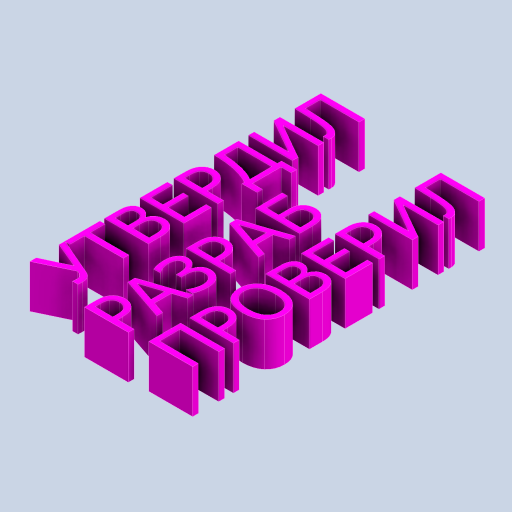
# Autodesk Inventor part: форма
Saved by Autodesk Inventor 2024.2 (Build 282272000, 272)
## iProperties
Created: 2025-11-21
Part Number: форма
Material: Типовые
Document SubType Name: Modeling
Designer: katya_notebook
Density: 1 g/cm^3
Appearance: Пурпурный
Author: katya_notebook
Autodesk Inventor part; units mm, degrees
ref_plane "YZ Plane" through (0, 0, 0) normal (1, 0, 0) x (0, 1, 0)
ref_plane "XZ Plane" through (0, 0, 0) normal (0, 1, 0) x (-1, 0, 0)
ref_plane "XY Plane" through (0, 0, 0) normal (0, 0, 1) x (1, 0, 0)
sketch "Эскиз1" plane through (0, 0, 0) normal (0, 1, 0) x (-1, 0, 0)
  line L0 (9.1599, 8.3568) -> (4.9033, 8.3568)
  line L1 (4.9033, 8.3568) -> (4.9033, -6.3257)
  line L2 (4.9033, -6.3257) -> (9.1599, -6.3257)
  line L3 (9.1599, -6.3257) -> (9.1599, 8.3568)
  line L4 (4.9459, 8.3568) -> (-6.0548, 8.3568)
  line L5 (-6.0548, 8.3568) -> (-6.0548, -6.3257)
  line L6 (-6.0548, -6.3257) -> (4.9459, -6.3257)
  line L7 (4.9459, -6.3257) -> (4.9459, 8.3568)
  line L8 (9.1599, -6.6362) -> (4.9033, -6.6362)
  line L9 (4.9033, -6.6362) -> (4.9033, -20.9369)
  line L10 (4.9033, -20.9369) -> (9.1599, -20.9369)
  line L11 (9.1599, -20.9369) -> (9.1599, -6.6362)
  line L12 (-6.0548, -6.2544) -> (-6.0548, -20.9369)
  line L13 (4.9459, -20.9369) -> (4.9459, -6.6362)
  line L14 (5.8791, -12.5357) -> (5.8791, 8.135)
  line L15 (4.9033, 7.9575) -> (4.9033, -6.7249)
  line L16 (4.9033, -6.7249) -> (9.1599, -6.7249)
  line L17 (9.1599, -6.7249) -> (9.1599, 8.3393)
  line L18 (-6.0548, 8.3393) -> (-6.0548, -6.7249)
  line L19 (4.9459, -6.3432) -> (4.9459, 8.3393)
  line L20 (0.9005, 8.7181) -> (0.9005, -5.6376) construction
  line L21 (0.9005, -5.6376) -> (-2.129, -5.6376) construction
  line L22 (-2.129, -5.6376) -> (-2.129, 8.7181) construction
  line L23 (-2.129, 8.7181) -> (0.9005, 8.7181) construction
  line L24 (-3.3858, 8.5472) -> (-3.3858, -12.3442) construction
  line L25 (-3.3858, -12.3442) -> (-5.6716, -12.3442) construction
  line L26 (-5.6716, -12.3442) -> (-5.6716, 8.5472) construction
  line L27 (-5.6716, 8.5472) -> (-3.3858, 8.5472) construction
  line L28 (5.4799, 7.5583) -> (5.4799, -12.9478) construction
  line L29 (5.4799, -12.9478) -> (1.7428, -12.9478) construction
  line L30 (1.7428, -12.9478) -> (1.7428, 7.5583) construction
  line L31 (1.7428, 7.5583) -> (5.4799, 7.5583) construction
  line L32 (5.4799, 5.1204) -> (2.9136, 6.227)
  spline S0 degree 2 poles (2.9136, 6.227) (2.7505, 6.2961) (2.5554, 6.469) (2.506, 6.5629) knots 0 0 0 1 2 2 2
  spline S1 degree 2 poles (2.506, 6.5629) (2.4541, 6.6592) (2.422, 6.8395) (2.422, 6.9334) knots 0 0 0 1 2 2 2
  spline S2 degree 2 poles (2.422, 6.9334) (2.422, 7.0149) (2.4294, 7.2372) (2.4319, 7.2669) knots 0 0 0 1 2 2 2
  line L33 (2.4319, 7.2669) -> (2.8123, 7.2669)
  line L34 (2.8123, 7.2669) -> (2.8123, 7.2372)
  spline S3 degree 2 poles (2.8123, 7.2372) (2.8073, 7.2076) (2.7975, 7.0816) (2.7975, 6.9853) knots 0 0 0 1 2 2 2
  spline S4 degree 2 poles (2.7975, 6.9853) (2.7975, 6.9408) (2.8073, 6.8173) (2.832, 6.7654) knots 0 0 0 1 2 2 2
  spline S5 degree 2 poles (2.832, 6.7654) (2.8617, 6.7062) (2.9555, 6.6024) (3.0618, 6.5604) knots 0 0 0 1 2 2 2
  line L35 (3.0618, 6.5604) -> (3.2223, 6.4888)
  line L36 (3.2223, 6.4888) -> (5.4799, 7.5608)
  line L37 (5.4799, 7.5608) -> (5.4799, 7.1112)
  line L38 (5.4799, 7.1112) -> (3.6867, 6.2838)
  line L39 (3.6867, 6.2838) -> (5.4799, 5.5378)
  line L40 (5.4799, 5.5378) -> (5.4799, 5.1204)
  line L41 (2.4319, 4.1275) -> (5.1193, 4.1275)
  line L42 (5.1193, 4.1275) -> (5.1193, 5.15)
  line L43 (5.1193, 5.15) -> (5.4799, 5.15)
  line L44 (5.4799, 5.15) -> (5.4799, 2.6998)
  line L45 (5.4799, 2.6998) -> (5.1193, 2.6998)
  line L46 (5.1193, 2.6998) -> (5.1193, 3.7224)
  line L47 (5.1193, 3.7224) -> (2.4319, 3.7224)
  line L48 (2.4319, 3.7224) -> (2.4319, 4.1275)
  spline S6 degree 2 poles (3.368, 0.3236) (3.1408, 0.3236) (2.7925, 0.4965) (2.6789, 0.6398) knots 0 0 0 1 2 2 2
  spline S7 degree 2 poles (2.6789, 0.6398) (2.5455, 0.8127) (2.4319, 1.2054) (2.4319, 1.5167) knots 0 0 0 1 2 2 2
  line L49 (2.4319, 1.5167) -> (2.4319, 2.391)
  line L50 (2.4319, 2.391) -> (5.4799, 2.391)
  line L51 (5.4799, 2.391) -> (5.4799, 1.5833)
  spline S8 degree 2 poles (5.4799, 1.5833) (5.4799, 1.2573) (5.4379, 0.9313) (5.3564, 0.7831) knots 0 0 0 1 2 2 2
  spline S9 degree 2 poles (5.3564, 0.7831) (5.27, 0.6176) (4.9859, 0.4669) (4.7932, 0.4669) knots 0 0 0 1 2 2 2
  spline S10 degree 2 poles (4.7932, 0.4669) (4.5783, 0.4669) (4.2375, 0.6941) (4.1412, 0.8942) knots 0 0 0 1 2 2 2
  line L52 (4.1412, 0.8942) -> (4.1263, 0.8942)
  spline S11 degree 2 poles (4.1263, 0.8942) (4.0522, 0.6225) (3.6595, 0.3236) (3.368, 0.3236) knots 0 0 0 1 2 2 2
  spline S12 degree 2 poles (3.3507, 0.746) (3.5236, 0.746) (3.746, 0.8448) (3.825, 0.993) knots 0 0 0 1 2 2 2
  spline S13 degree 2 poles (3.825, 0.993) (3.8744, 1.0893) (3.904, 1.3166) (3.904, 1.5265) knots 0 0 0 1 2 2 2
  line L53 (3.904, 1.5265) -> (3.904, 1.986)
  line L54 (3.904, 1.986) -> (2.7777, 1.986)
  line L55 (2.7777, 1.986) -> (2.7777, 1.6574)
  spline S14 degree 2 poles (2.7777, 1.6574) (2.7777, 1.3907) (2.8271, 1.0844) (2.9061, 0.9658) knots 0 0 0 1 2 2 2
  spline S15 degree 2 poles (2.9061, 0.9658) (2.9877, 0.8522) (3.1902, 0.746) (3.3507, 0.746) knots 0 0 0 1 2 2 2
  spline S16 degree 2 poles (4.7364, 0.8893) (4.8451, 0.8893) (5.0081, 0.9634) (5.0551, 1.0449) knots 0 0 0 1 2 2 2
  spline S17 degree 2 poles (5.0551, 1.0449) (5.1094, 1.1437) (5.1341, 1.3833) (5.1341, 1.5982) knots 0 0 0 1 2 2 2
  line L56 (5.1341, 1.5982) -> (5.1341, 1.986)
  line L57 (5.1341, 1.986) -> (4.2424, 1.986)
  line L58 (4.2424, 1.986) -> (4.2424, 1.5265)
  spline S18 degree 2 poles (4.2424, 1.5265) (4.2424, 1.3363) (4.2819, 1.156) (4.3437, 1.0597) knots 0 0 0 1 2 2 2
  spline S19 degree 2 poles (4.3437, 1.0597) (4.403, 0.9658) (4.5932, 0.8893) (4.7364, 0.8893) knots 0 0 0 1 2 2 2
  line L59 (2.4319, -0.079) -> (5.4799, -0.079)
  line L60 (5.4799, -0.079) -> (5.4799, -1.9858)
  line L61 (5.4799, -1.9858) -> (5.1193, -1.9858)
  line L62 (5.1193, -1.9858) -> (5.1193, -0.4841)
  line L63 (5.1193, -0.4841) -> (4.2844, -0.4841)
  line L64 (4.2844, -0.4841) -> (4.2844, -1.8846)
  line L65 (4.2844, -1.8846) -> (3.9238, -1.8846)
  line L66 (3.9238, -1.8846) -> (3.9238, -0.4841)
  line L67 (3.9238, -0.4841) -> (2.7925, -0.4841)
  line L68 (2.7925, -0.4841) -> (2.7925, -1.9858)
  line L69 (2.7925, -1.9858) -> (2.4319, -1.9858)
  line L70 (2.4319, -1.9858) -> (2.4319, -0.079)
  spline S20 degree 2 poles (4.5611, -4.357) (4.3635, -4.357) (4.0078, -4.2163) (3.8843, -4.0903) knots 0 0 0 1 2 2 2
  spline S21 degree 2 poles (3.8843, -4.0903) (3.7287, -3.9322) (3.5681, -3.5049) (3.5681, -3.1788) knots 0 0 0 1 2 2 2
  line L71 (3.5681, -3.1788) -> (3.5681, -2.8355)
  line L72 (3.5681, -2.8355) -> (2.4319, -2.8355)
  line L73 (2.4319, -2.8355) -> (2.4319, -2.4304)
  line L74 (2.4319, -2.4304) -> (5.4799, -2.4304)
  line L75 (5.4799, -2.4304) -> (5.4799, -3.1961)
  spline S22 degree 2 poles (5.4799, -3.1961) (5.4799, -3.4678) (5.391, -3.8482) (5.2897, -3.994) knots 0 0 0 1 2 2 2
  spline S23 degree 2 poles (5.2897, -3.994) (5.1736, -4.1644) (4.8155, -4.357) (4.5611, -4.357) knots 0 0 0 1 2 2 2
  spline S24 degree 2 poles (4.5487, -3.9347) (4.7068, -3.9347) (4.939, -3.826) (5.0131, -3.7148) knots 0 0 0 1 2 2 2
  spline S25 degree 2 poles (5.0131, -3.7148) (5.0773, -3.6185) (5.1292, -3.3616) (5.1292, -3.1714) knots 0 0 0 1 2 2 2
  line L76 (5.1292, -3.1714) -> (5.1292, -2.8355)
  line L77 (5.1292, -2.8355) -> (3.9139, -2.8355)
  line L78 (3.9139, -2.8355) -> (3.9139, -3.1122)
  spline S26 degree 2 poles (3.9139, -3.1122) (3.9139, -3.3592) (3.993, -3.663) (4.0967, -3.7618) knots 0 0 0 1 2 2 2
  spline S27 degree 2 poles (4.0967, -3.7618) (4.1881, -3.8532) (4.403, -3.9347) (4.5487, -3.9347) knots 0 0 0 1 2 2 2
  line L79 (1.7428, -7.2173) -> (1.7428, -6.832)
  line L80 (1.7428, -6.832) -> (2.4393, -6.832)
  line L81 (2.4393, -6.832) -> (2.4393, -4.856)
  line L82 (2.4393, -4.856) -> (1.7428, -4.856)
  line L83 (1.7428, -4.856) -> (1.7428, -4.4707)
  line L84 (1.7428, -4.4707) -> (2.7901, -4.4707)
  line L85 (2.7901, -4.4707) -> (2.7901, -4.6362)
  spline S28 degree 2 poles (2.7901, -4.6362) (3.2272, -4.9029) (4.6426, -5.2265) (5.4799, -5.2265) knots 0 0 0 1 2 2 2
  line L86 (5.4799, -5.2265) -> (5.4799, -6.9283)
  line L87 (5.4799, -6.9283) -> (2.7901, -6.9283)
  line L88 (2.7901, -6.9283) -> (2.7901, -7.2173)
  line L89 (2.7901, -7.2173) -> (1.7428, -7.2173)
  line L90 (2.7901, -6.5232) -> (5.1292, -6.5232)
  line L91 (5.1292, -6.5232) -> (5.1292, -5.6044)
  spline S29 degree 2 poles (5.1292, -5.6044) (4.3882, -5.5748) (3.1828, -5.266) (2.7901, -5.0264) knots 0 0 0 1 2 2 2
  line L92 (2.7901, -5.0264) -> (2.7901, -6.5232)
  line L93 (2.4319, -9.7985) -> (2.4319, -9.3934)
  line L94 (2.4319, -9.3934) -> (4.8525, -9.3934)
  line L95 (4.8525, -9.3934) -> (2.4319, -8.0176)
  line L96 (2.4319, -8.0176) -> (2.4319, -7.6076)
  line L97 (2.4319, -7.6076) -> (5.4799, -7.6076)
  line L98 (5.4799, -7.6076) -> (5.4799, -8.0127)
  line L99 (5.4799, -8.0127) -> (3.0988, -8.0127)
  line L100 (3.0988, -8.0127) -> (5.4799, -9.3687)
  line L101 (5.4799, -9.3687) -> (5.4799, -9.7985)
  line L102 (5.4799, -9.7985) -> (2.4319, -9.7985)
  line L103 (2.4319, -12.639) -> (2.4319, -12.2339)
  line L104 (2.4319, -12.2339) -> (5.1193, -12.2339)
  line L105 (5.1193, -12.2339) -> (5.1193, -11.2064)
  spline S30 degree 2 poles (5.1193, -11.2064) (4.8871, -11.2015) (4.4474, -11.1792) (4.2745, -11.1743) knots 0 0 0 1 2 2 2
  spline S31 degree 2 poles (4.2745, -11.1743) (3.8423, -11.157) (3.2791, -11.0854) (3.0889, -11.0286) knots 0 0 0 1 2 2 2
  spline S32 degree 2 poles (3.0889, -11.0286) (2.9012, -10.9717) (2.6715, -10.8235) (2.5949, -10.7346) knots 0 0 0 1 2 2 2
  spline S33 degree 2 poles (2.5949, -10.7346) (2.5109, -10.6432) (2.427, -10.4308) (2.427, -10.2925) knots 0 0 0 1 2 2 2
  spline S34 degree 2 poles (2.427, -10.2925) (2.427, -10.2505) (2.4319, -10.1616) (2.4319, -10.1369) knots 0 0 0 1 2 2 2
  line L106 (2.4319, -10.1369) -> (2.8246, -10.1369)
  line L107 (2.8246, -10.1369) -> (2.8246, -10.1665)
  spline S35 degree 2 poles (2.8246, -10.1665) (2.8222, -10.1863) (2.8197, -10.2159) (2.8197, -10.2431) knots 0 0 0 1 2 2 2
  spline S36 degree 2 poles (2.8197, -10.2431) (2.8197, -10.3172) (2.8642, -10.4432) (2.9111, -10.4901) knots 0 0 0 1 2 2 2
  spline S37 degree 2 poles (2.9111, -10.4901) (3.0494, -10.6284) (3.7509, -10.7569) (4.3437, -10.784) knots 0 0 0 1 2 2 2
  spline S38 degree 2 poles (4.3437, -10.784) (4.5438, -10.7939) (5.2033, -10.8161) (5.4799, -10.8235) knots 0 0 0 1 2 2 2
  line L108 (5.4799, -10.8235) -> (5.4799, -12.639)
  line L109 (5.4799, -12.639) -> (2.4319, -12.639)
  spline S39 degree 2 poles (-0.0727, 6.4827) (-0.2703, 6.4827) (-0.626, 6.6235) (-0.7495, 6.7495) knots 0 0 0 1 2 2 2
  spline S40 degree 2 poles (-0.7495, 6.7495) (-0.9051, 6.9076) (-1.0657, 7.3349) (-1.0657, 7.6609) knots 0 0 0 1 2 2 2
  line L110 (-1.0657, 7.6609) -> (-1.0657, 8.0043)
  line L111 (-1.0657, 8.0043) -> (-2.2019, 8.0043)
  line L112 (-2.2019, 8.0043) -> (-2.2019, 8.4093)
  line L113 (-2.2019, 8.4093) -> (0.8461, 8.4093)
  line L114 (0.8461, 8.4093) -> (0.8461, 7.6436)
  spline S41 degree 2 poles (0.8461, 7.6436) (0.8461, 7.3719) (0.7572, 6.9916) (0.6559, 6.8458) knots 0 0 0 1 2 2 2
  spline S42 degree 2 poles (0.6559, 6.8458) (0.5398, 6.6754) (0.1817, 6.4827) (-0.0727, 6.4827) knots 0 0 0 1 2 2 2
  spline S43 degree 2 poles (-0.0851, 6.9051) (0.073, 6.9051) (0.3052, 7.0138) (0.3793, 7.1249) knots 0 0 0 1 2 2 2
  spline S44 degree 2 poles (0.3793, 7.1249) (0.4435, 7.2213) (0.4954, 7.4782) (0.4954, 7.6683) knots 0 0 0 1 2 2 2
  line L115 (0.4954, 7.6683) -> (0.4954, 8.0043)
  line L116 (0.4954, 8.0043) -> (-0.7199, 8.0043)
  line L117 (-0.7199, 8.0043) -> (-0.7199, 7.7276)
  spline S45 degree 2 poles (-0.7199, 7.7276) (-0.7199, 7.4806) (-0.6408, 7.1768) (-0.5371, 7.078) knots 0 0 0 1 2 2 2
  spline S46 degree 2 poles (-0.5371, 7.078) (-0.4457, 6.9866) (-0.2308, 6.9051) (-0.0851, 6.9051) knots 0 0 0 1 2 2 2
  line L118 (-2.2019, 6.4259) -> (0.8461, 5.3984)
  line L119 (0.8461, 5.3984) -> (0.8461, 4.8995)
  line L120 (0.8461, 4.8995) -> (-2.2019, 3.8719)
  line L121 (-2.2019, 3.8719) -> (-2.2019, 4.2992)
  line L122 (-2.2019, 4.2992) -> (-1.3497, 4.5759)
  line L123 (-1.3497, 4.5759) -> (-1.3497, 5.7393)
  line L124 (-1.3497, 5.7393) -> (-2.2019, 6.0159)
  line L125 (-2.2019, 6.0159) -> (-2.2019, 6.4259)
  line L126 (-1.0039, 4.687) -> (0.4312, 5.1588)
  line L127 (0.4312, 5.1588) -> (-1.0039, 5.6281)
  line L128 (-1.0039, 5.6281) -> (-1.0039, 4.687)
  spline S47 degree 2 poles (-0.7322, 2.0071) (-0.8211, 1.9058) (-1.0854, 1.7724) (-1.2929, 1.7724) knots 0 0 0 1 2 2 2
  spline S48 degree 2 poles (-1.2929, 1.7724) (-1.4979, 1.7724) (-1.8462, 1.9354) (-1.9771, 2.0787) knots 0 0 0 1 2 2 2
  spline S49 degree 2 poles (-1.9771, 2.0787) (-2.113, 2.2269) (-2.2562, 2.6592) (-2.2562, 2.9259) knots 0 0 0 1 2 2 2
  spline S50 degree 2 poles (-2.2562, 2.9259) (-2.2562, 3.21) (-2.1426, 3.6842) (-2.0833, 3.8275) knots 0 0 0 1 2 2 2
  line L129 (-2.0833, 3.8275) -> (-1.6288, 3.8275)
  line L130 (-1.6288, 3.8275) -> (-1.6288, 3.7978)
  spline S51 degree 2 poles (-1.6288, 3.7978) (-1.7375, 3.6348) (-1.903, 3.168) (-1.903, 2.9333) knots 0 0 0 1 2 2 2
  spline S52 degree 2 poles (-1.903, 2.9333) (-1.903, 2.7851) (-1.824, 2.4887) (-1.7326, 2.3874) knots 0 0 0 1 2 2 2
  spline S53 degree 2 poles (-1.7326, 2.3874) (-1.6437, 2.2886) (-1.4337, 2.1948) (-1.2732, 2.1948) knots 0 0 0 1 2 2 2
  spline S54 degree 2 poles (-1.2732, 2.1948) (-1.1175, 2.1948) (-0.9051, 2.3059) (-0.8409, 2.4097) knots 0 0 0 1 2 2 2
  spline S55 degree 2 poles (-0.8409, 2.4097) (-0.7742, 2.5085) (-0.7199, 2.7876) (-0.7199, 2.9457) knots 0 0 0 1 2 2 2
  line L131 (-0.7199, 2.9457) -> (-0.7199, 3.2643)
  line L132 (-0.7199, 3.2643) -> (-0.379, 3.2643)
  line L133 (-0.379, 3.2643) -> (-0.379, 2.9852)
  spline S56 degree 2 poles (-0.379, 2.9852) (-0.379, 2.6641) (-0.1197, 2.2714) (0.1273, 2.2714) knots 0 0 0 1 2 2 2
  spline S57 degree 2 poles (0.1273, 2.2714) (0.241, 2.2714) (0.4015, 2.3677) (0.4534, 2.4541) knots 0 0 0 1 2 2 2
  spline S58 degree 2 poles (0.4534, 2.4541) (0.5077, 2.5505) (0.5472, 2.7629) (0.5472, 2.8864) knots 0 0 0 1 2 2 2
  spline S59 degree 2 poles (0.5472, 2.8864) (0.5472, 3.0173) (0.488, 3.2717) (0.4435, 3.3829) knots 0 0 0 1 2 2 2
  spline S60 degree 2 poles (0.4435, 3.3829) (0.4015, 3.4891) (0.3077, 3.6496) (0.2755, 3.699) knots 0 0 0 1 2 2 2
  line L134 (0.2755, 3.699) -> (0.2755, 3.7262)
  line L135 (0.2755, 3.7262) -> (0.7251, 3.7262)
  spline S61 degree 2 poles (0.7251, 3.7262) (0.7893, 3.5879) (0.9005, 3.1087) (0.9005, 2.8765) knots 0 0 0 1 2 2 2
  spline S62 degree 2 poles (0.9005, 2.8765) (0.9005, 2.6419) (0.8214, 2.301) (0.73, 2.1602) knots 0 0 0 1 2 2 2
  spline S63 degree 2 poles (0.73, 2.1602) (0.6312, 2.0071) (0.3571, 1.8539) (0.1693, 1.8539) knots 0 0 0 1 2 2 2
  spline S64 degree 2 poles (0.1693, 1.8539) (-0.0777, 1.8539) (-0.4457, 2.1824) (-0.505, 2.4492) knots 0 0 0 1 2 2 2
  line L136 (-0.505, 2.4492) -> (-0.5346, 2.4492)
  spline S65 degree 2 poles (-0.5346, 2.4492) (-0.5544, 2.3479) (-0.6482, 2.1083) (-0.7322, 2.0071) knots 0 0 0 1 2 2 2
  spline S66 degree 2 poles (-0.0727, -0.5766) (-0.2703, -0.5766) (-0.626, -0.4358) (-0.7495, -0.3098) knots 0 0 0 1 2 2 2
  spline S67 degree 2 poles (-0.7495, -0.3098) (-0.9051, -0.1517) (-1.0657, 0.2756) (-1.0657, 0.6016) knots 0 0 0 1 2 2 2
  line L137 (-1.0657, 0.6016) -> (-1.0657, 0.945)
  line L138 (-1.0657, 0.945) -> (-2.2019, 0.945)
  line L139 (-2.2019, 0.945) -> (-2.2019, 1.35)
  line L140 (-2.2019, 1.35) -> (0.8461, 1.35)
  line L141 (0.8461, 1.35) -> (0.8461, 0.5843)
  spline S68 degree 2 poles (0.8461, 0.5843) (0.8461, 0.3126) (0.7572, -0.0677) (0.6559, -0.2135) knots 0 0 0 1 2 2 2
  spline S69 degree 2 poles (0.6559, -0.2135) (0.5398, -0.3839) (0.1817, -0.5766) (-0.0727, -0.5766) knots 0 0 0 1 2 2 2
  spline S70 degree 2 poles (-0.0851, -0.1542) (0.073, -0.1542) (0.3052, -0.0455) (0.3793, 0.0656) knots 0 0 0 1 2 2 2
  spline S71 degree 2 poles (0.3793, 0.0656) (0.4435, 0.162) (0.4954, 0.4188) (0.4954, 0.609) knots 0 0 0 1 2 2 2
  line L142 (0.4954, 0.609) -> (0.4954, 0.945)
  line L143 (0.4954, 0.945) -> (-0.7199, 0.945)
  line L144 (-0.7199, 0.945) -> (-0.7199, 0.6683)
  spline S72 degree 2 poles (-0.7199, 0.6683) (-0.7199, 0.4213) (-0.6408, 0.1175) (-0.5371, 0.0187) knots 0 0 0 1 2 2 2
  spline S73 degree 2 poles (-0.5371, 0.0187) (-0.4457, -0.0727) (-0.2308, -0.1542) (-0.0851, -0.1542) knots 0 0 0 1 2 2 2
  line L145 (-2.2019, -0.6334) -> (0.8461, -1.6609)
  line L146 (0.8461, -1.6609) -> (0.8461, -2.1599)
  line L147 (0.8461, -2.1599) -> (-2.2019, -3.1874)
  line L148 (-2.2019, -3.1874) -> (-2.2019, -2.7601)
  line L149 (-2.2019, -2.7601) -> (-1.3497, -2.4834)
  line L150 (-1.3497, -2.4834) -> (-1.3497, -1.32)
  line L151 (-1.3497, -1.32) -> (-2.2019, -1.0434)
  line L152 (-2.2019, -1.0434) -> (-2.2019, -0.6334)
  line L153 (-1.0039, -2.3723) -> (0.4312, -1.9005)
  line L154 (0.4312, -1.9005) -> (-1.0039, -1.4312)
  line L155 (-1.0039, -1.4312) -> (-1.0039, -2.3723)
  spline S74 degree 2 poles (-1.2583, -5.5512) (-1.4782, -5.5512) (-1.8388, -5.3783) (-1.9524, -5.235) knots 0 0 0 1 2 2 2
  spline S75 degree 2 poles (-1.9524, -5.235) (-2.0883, -5.0621) (-2.2019, -4.6694) (-2.2019, -4.3582) knots 0 0 0 1 2 2 2
  line L156 (-2.2019, -4.3582) -> (-2.2019, -3.4764)
  line L157 (-2.2019, -3.4764) -> (0.8461, -3.4764)
  line L158 (0.8461, -3.4764) -> (0.8461, -5.3314)
  line L159 (0.8461, -5.3314) -> (0.4855, -5.3314)
  line L160 (0.4855, -5.3314) -> (0.4855, -3.8815)
  line L161 (0.4855, -3.8815) -> (-0.3494, -3.8815)
  line L162 (-0.3494, -3.8815) -> (-0.3494, -4.3705)
  spline S76 degree 2 poles (-0.3494, -4.3705) (-0.3494, -4.6817) (-0.421, -5.0745) (-0.5569, -5.2474) knots 0 0 0 1 2 2 2
  spline S77 degree 2 poles (-0.5569, -5.2474) (-0.6779, -5.403) (-1.0336, -5.5512) (-1.2583, -5.5512) knots 0 0 0 1 2 2 2
  spline S78 degree 2 poles (-1.2657, -5.1288) (-1.1126, -5.1288) (-0.8804, -5.0275) (-0.8088, -4.9189) knots 0 0 0 1 2 2 2
  spline S79 degree 2 poles (-0.8088, -4.9189) (-0.7322, -4.8077) (-0.7001, -4.5113) (-0.7001, -4.2445) knots 0 0 0 1 2 2 2
  line L163 (-0.7001, -4.2445) -> (-0.7001, -3.8815)
  line L164 (-0.7001, -3.8815) -> (-1.8561, -3.8815)
  line L165 (-1.8561, -3.8815) -> (-1.8561, -4.2347)
  spline S80 degree 2 poles (-1.8561, -4.2347) (-1.8561, -4.5064) (-1.8017, -4.8003) (-1.7276, -4.909) knots 0 0 0 1 2 2 2
  spline S81 degree 2 poles (-1.7276, -4.909) (-1.6486, -5.0251) (-1.4337, -5.1288) (-1.2657, -5.1288) knots 0 0 0 1 2 2 2
  line L166 (-6.498, 6.0254) -> (-6.498, 6.4304)
  line L167 (-6.498, 6.4304) -> (-3.8107, 6.4304)
  line L168 (-3.8107, 6.4304) -> (-3.8107, 7.8334)
  line L169 (-3.8107, 7.8334) -> (-6.498, 7.8334)
  line L170 (-6.498, 7.8334) -> (-6.498, 8.2385)
  line L171 (-6.498, 8.2385) -> (-3.45, 8.2385)
  line L172 (-3.45, 8.2385) -> (-3.45, 6.0254)
  line L173 (-3.45, 6.0254) -> (-6.498, 6.0254)
  spline S82 degree 2 poles (-4.3689, 3.4812) (-4.5665, 3.4812) (-4.9222, 3.622) (-5.0457, 3.748) knots 0 0 0 1 2 2 2
  spline S83 degree 2 poles (-5.0457, 3.748) (-5.2013, 3.9061) (-5.3618, 4.3334) (-5.3618, 4.6594) knots 0 0 0 1 2 2 2
  line L174 (-5.3618, 4.6594) -> (-5.3618, 5.0028)
  line L175 (-5.3618, 5.0028) -> (-6.498, 5.0028)
  line L176 (-6.498, 5.0028) -> (-6.498, 5.4079)
  line L177 (-6.498, 5.4079) -> (-3.45, 5.4079)
  line L178 (-3.45, 5.4079) -> (-3.45, 4.6421)
  spline S84 degree 2 poles (-3.45, 4.6421) (-3.45, 4.3704) (-3.539, 3.9901) (-3.6402, 3.8443) knots 0 0 0 1 2 2 2
  spline S85 degree 2 poles (-3.6402, 3.8443) (-3.7563, 3.6739) (-4.1145, 3.4812) (-4.3689, 3.4812) knots 0 0 0 1 2 2 2
  spline S86 degree 2 poles (-4.3812, 3.9036) (-4.2232, 3.9036) (-3.991, 4.0123) (-3.9169, 4.1234) knots 0 0 0 1 2 2 2
  spline S87 degree 2 poles (-3.9169, 4.1234) (-3.8526, 4.2198) (-3.8008, 4.4767) (-3.8008, 4.6668) knots 0 0 0 1 2 2 2
  line L179 (-3.8008, 4.6668) -> (-3.8008, 5.0028)
  line L180 (-3.8008, 5.0028) -> (-5.016, 5.0028)
  line L181 (-5.016, 5.0028) -> (-5.016, 4.7261)
  spline S88 degree 2 poles (-5.016, 4.7261) (-5.016, 4.4791) (-4.937, 4.1753) (-4.8332, 4.0765) knots 0 0 0 1 2 2 2
  spline S89 degree 2 poles (-4.8332, 4.0765) (-4.7419, 3.9851) (-4.527, 3.9036) (-4.3812, 3.9036) knots 0 0 0 1 2 2 2
  spline S90 degree 2 poles (-3.7983, 0.9396) (-4.0008, 0.7667) (-4.5937, 0.574) (-4.974, 0.574) knots 0 0 0 1 2 2 2
  spline S91 degree 2 poles (-4.974, 0.574) (-5.3445, 0.574) (-5.9448, 0.7618) (-6.1473, 0.9396) knots 0 0 0 1 2 2 2
  spline S92 degree 2 poles (-6.1473, 0.9396) (-6.3597, 1.1273) (-6.5623, 1.6238) (-6.5623, 1.9227) knots 0 0 0 1 2 2 2
  spline S93 degree 2 poles (-6.5623, 1.9227) (-6.5623, 2.2314) (-6.3523, 2.7254) (-6.1473, 2.9057) knots 0 0 0 1 2 2 2
  spline S94 degree 2 poles (-6.1473, 2.9057) (-5.9448, 3.0811) (-5.3495, 3.2688) (-4.974, 3.2688) knots 0 0 0 1 2 2 2
  spline S95 degree 2 poles (-4.974, 3.2688) (-4.5912, 3.2688) (-4.0083, 3.0786) (-3.7983, 2.9033) knots 0 0 0 1 2 2 2
  spline S96 degree 2 poles (-3.7983, 2.9033) (-3.5958, 2.7254) (-3.3858, 2.2289) (-3.3858, 1.9227) knots 0 0 0 1 2 2 2
  spline S97 degree 2 poles (-3.3858, 1.9227) (-3.3858, 1.6114) (-3.6032, 1.1125) (-3.7983, 0.9396) knots 0 0 0 1 2 2 2
  spline S98 degree 2 poles (-4.974, 0.9964) (-4.6727, 0.9964) (-4.2059, 1.1273) (-4.0527, 1.2459) knots 0 0 0 1 2 2 2
  spline S99 degree 2 poles (-4.0527, 1.2459) (-3.8946, 1.3669) (-3.7366, 1.7078) (-3.7366, 1.9202) knots 0 0 0 1 2 2 2
  spline S100 degree 2 poles (-3.7366, 1.9202) (-3.7366, 2.14) (-3.8897, 2.471) (-4.0527, 2.597) knots 0 0 0 1 2 2 2
  spline S101 degree 2 poles (-4.0527, 2.597) (-4.2083, 2.718) (-4.6776, 2.8464) (-4.974, 2.8464) knots 0 0 0 1 2 2 2
  spline S102 degree 2 poles (-4.974, 2.8464) (-5.5743, 2.8464) (-6.2115, 2.3426) (-6.2115, 1.9202) knots 0 0 0 1 2 2 2
  spline S103 degree 2 poles (-6.2115, 1.9202) (-6.2115, 1.4978) (-5.5743, 0.9964) (-4.974, 0.9964) knots 0 0 0 1 2 2 2
  spline S104 degree 2 poles (-5.5619, -1.938) (-5.7891, -1.938) (-6.1374, -1.7651) (-6.251, -1.6218) knots 0 0 0 1 2 2 2
  spline S105 degree 2 poles (-6.251, -1.6218) (-6.3844, -1.4489) (-6.498, -1.0562) (-6.498, -0.745) knots 0 0 0 1 2 2 2
  line L182 (-6.498, -0.745) -> (-6.498, 0.1294)
  line L183 (-6.498, 0.1294) -> (-3.45, 0.1294)
  line L184 (-3.45, 0.1294) -> (-3.45, -0.6783)
  spline S106 degree 2 poles (-3.45, -0.6783) (-3.45, -1.0043) (-3.492, -1.3304) (-3.5735, -1.4786) knots 0 0 0 1 2 2 2
  spline S107 degree 2 poles (-3.5735, -1.4786) (-3.66, -1.644) (-3.944, -1.7947) (-4.1367, -1.7947) knots 0 0 0 1 2 2 2
  spline S108 degree 2 poles (-4.1367, -1.7947) (-4.3516, -1.7947) (-4.6925, -1.5675) (-4.7888, -1.3674) knots 0 0 0 1 2 2 2
  line L185 (-4.7888, -1.3674) -> (-4.8036, -1.3674)
  spline S109 degree 2 poles (-4.8036, -1.3674) (-4.8777, -1.6391) (-5.2704, -1.938) (-5.5619, -1.938) knots 0 0 0 1 2 2 2
  spline S110 degree 2 poles (-5.5792, -1.5156) (-5.4063, -1.5156) (-5.184, -1.4168) (-5.1049, -1.2686) knots 0 0 0 1 2 2 2
  spline S111 degree 2 poles (-5.1049, -1.2686) (-5.0555, -1.1723) (-5.0259, -0.945) (-5.0259, -0.7351) knots 0 0 0 1 2 2 2
  line L186 (-5.0259, -0.7351) -> (-5.0259, -0.2757)
  line L187 (-5.0259, -0.2757) -> (-6.1522, -0.2757)
  line L188 (-6.1522, -0.2757) -> (-6.1522, -0.6042)
  spline S112 degree 2 poles (-6.1522, -0.6042) (-6.1522, -0.8709) (-6.1028, -1.1772) (-6.0238, -1.2958) knots 0 0 0 1 2 2 2
  spline S113 degree 2 poles (-6.0238, -1.2958) (-5.9423, -1.4094) (-5.7397, -1.5156) (-5.5792, -1.5156) knots 0 0 0 1 2 2 2
  spline S114 degree 2 poles (-4.1935, -1.3723) (-4.0848, -1.3723) (-3.9218, -1.2982) (-3.8749, -1.2167) knots 0 0 0 1 2 2 2
  spline S115 degree 2 poles (-3.8749, -1.2167) (-3.8205, -1.1179) (-3.7958, -0.8783) (-3.7958, -0.6634) knots 0 0 0 1 2 2 2
  line L189 (-3.7958, -0.6634) -> (-3.7958, -0.2757)
  line L190 (-3.7958, -0.2757) -> (-4.6875, -0.2757)
  line L191 (-4.6875, -0.2757) -> (-4.6875, -0.7351)
  spline S116 degree 2 poles (-4.6875, -0.7351) (-4.6875, -0.9253) (-4.648, -1.1056) (-4.5862, -1.2019) knots 0 0 0 1 2 2 2
  spline S117 degree 2 poles (-4.5862, -1.2019) (-4.527, -1.2958) (-4.3368, -1.3723) (-4.1935, -1.3723) knots 0 0 0 1 2 2 2
  line L192 (-6.498, -2.3406) -> (-3.45, -2.3406)
  line L193 (-3.45, -2.3406) -> (-3.45, -4.2474)
  line L194 (-3.45, -4.2474) -> (-3.8107, -4.2474)
  line L195 (-3.8107, -4.2474) -> (-3.8107, -2.7457)
  line L196 (-3.8107, -2.7457) -> (-4.6455, -2.7457)
  line L197 (-4.6455, -2.7457) -> (-4.6455, -4.1462)
  line L198 (-4.6455, -4.1462) -> (-5.0061, -4.1462)
  line L199 (-5.0061, -4.1462) -> (-5.0061, -2.7457)
  line L200 (-5.0061, -2.7457) -> (-6.1374, -2.7457)
  line L201 (-6.1374, -2.7457) -> (-6.1374, -4.2474)
  line L202 (-6.1374, -4.2474) -> (-6.498, -4.2474)
  line L203 (-6.498, -4.2474) -> (-6.498, -2.3406)
  spline S118 degree 2 poles (-4.3689, -6.6187) (-4.5665, -6.6187) (-4.9222, -6.4779) (-5.0457, -6.3519) knots 0 0 0 1 2 2 2
  spline S119 degree 2 poles (-5.0457, -6.3519) (-5.2013, -6.1938) (-5.3618, -5.7665) (-5.3618, -5.4405) knots 0 0 0 1 2 2 2
  line L204 (-5.3618, -5.4405) -> (-5.3618, -5.0971)
  line L205 (-5.3618, -5.0971) -> (-6.498, -5.0971)
  line L206 (-6.498, -5.0971) -> (-6.498, -4.692)
  line L207 (-6.498, -4.692) -> (-3.45, -4.692)
  line L208 (-3.45, -4.692) -> (-3.45, -5.4577)
  spline S120 degree 2 poles (-3.45, -5.4577) (-3.45, -5.7294) (-3.539, -6.1098) (-3.6402, -6.2556) knots 0 0 0 1 2 2 2
  spline S121 degree 2 poles (-3.6402, -6.2556) (-3.7563, -6.426) (-4.1145, -6.6187) (-4.3689, -6.6187) knots 0 0 0 1 2 2 2
  spline S122 degree 2 poles (-4.3812, -6.1963) (-4.2232, -6.1963) (-3.991, -6.0876) (-3.9169, -5.9765) knots 0 0 0 1 2 2 2
  spline S123 degree 2 poles (-3.9169, -5.9765) (-3.8526, -5.8801) (-3.8008, -5.6232) (-3.8008, -5.433) knots 0 0 0 1 2 2 2
  line L209 (-3.8008, -5.433) -> (-3.8008, -5.0971)
  line L210 (-3.8008, -5.0971) -> (-5.016, -5.0971)
  line L211 (-5.016, -5.0971) -> (-5.016, -5.3738)
  spline S124 degree 2 poles (-5.016, -5.3738) (-5.016, -5.6208) (-4.937, -5.9246) (-4.8332, -6.0234) knots 0 0 0 1 2 2 2
  spline S125 degree 2 poles (-4.8332, -6.0234) (-4.7419, -6.1148) (-4.527, -6.1963) (-4.3812, -6.1963) knots 0 0 0 1 2 2 2
  line L212 (-6.498, -9.1949) -> (-6.498, -8.7898)
  line L213 (-6.498, -8.7898) -> (-4.0774, -8.7898)
  line L214 (-4.0774, -8.7898) -> (-6.498, -7.414)
  line L215 (-6.498, -7.414) -> (-6.498, -7.004)
  line L216 (-6.498, -7.004) -> (-3.45, -7.004)
  line L217 (-3.45, -7.004) -> (-3.45, -7.4091)
  line L218 (-3.45, -7.4091) -> (-5.8311, -7.4091)
  line L219 (-5.8311, -7.4091) -> (-3.45, -8.7651)
  line L220 (-3.45, -8.7651) -> (-3.45, -9.1949)
  line L221 (-3.45, -9.1949) -> (-6.498, -9.1949)
  line L222 (-6.498, -12.0354) -> (-6.498, -11.6303)
  line L223 (-6.498, -11.6303) -> (-3.8107, -11.6303)
  line L224 (-3.8107, -11.6303) -> (-3.8107, -10.6028)
  spline S126 degree 2 poles (-3.8107, -10.6028) (-4.0428, -10.5979) (-4.4825, -10.5756) (-4.6554, -10.5707) knots 0 0 0 1 2 2 2
  spline S127 degree 2 poles (-4.6554, -10.5707) (-5.0877, -10.5534) (-5.6508, -10.4818) (-5.841, -10.425) knots 0 0 0 1 2 2 2
  spline S128 degree 2 poles (-5.841, -10.425) (-6.0287, -10.3681) (-6.2584, -10.2199) (-6.335, -10.131) knots 0 0 0 1 2 2 2
  spline S129 degree 2 poles (-6.335, -10.131) (-6.419, -10.0396) (-6.503, -9.8272) (-6.503, -9.6889) knots 0 0 0 1 2 2 2
  spline S130 degree 2 poles (-6.503, -9.6889) (-6.503, -9.6469) (-6.498, -9.558) (-6.498, -9.5333) knots 0 0 0 1 2 2 2
  line L225 (-6.498, -9.5333) -> (-6.1053, -9.5333)
  line L226 (-6.1053, -9.5333) -> (-6.1053, -9.5629)
  spline S131 degree 2 poles (-6.1053, -9.5629) (-6.1078, -9.5827) (-6.1102, -9.6123) (-6.1102, -9.6395) knots 0 0 0 1 2 2 2
  spline S132 degree 2 poles (-6.1102, -9.6395) (-6.1102, -9.7136) (-6.0658, -9.8396) (-6.0189, -9.8865) knots 0 0 0 1 2 2 2
  spline S133 degree 2 poles (-6.0189, -9.8865) (-5.8805, -10.0248) (-5.179, -10.1532) (-4.5862, -10.1804) knots 0 0 0 1 2 2 2
  spline S134 degree 2 poles (-4.5862, -10.1804) (-4.3862, -10.1903) (-3.7267, -10.2125) (-3.45, -10.2199) knots 0 0 0 1 2 2 2
  line L227 (-3.45, -10.2199) -> (-3.45, -12.0354)
  line L228 (-3.45, -12.0354) -> (-6.498, -12.0354)
  point P0 (0, 0)
  constraints: 40 end point, 9 parallel, 5 point on line, 3 horizontal, 3 perpendicular, 6 other
extrude "Выдавливание1" add sketch "Эскиз1" along normal blind 3 contours S132 S133 S134 L227 L228 L12 L223 L224 S126 S127 S128 | L12 S128 S129 S130 L225 L226 S131 S132 | L216 L217 L218 L219 L220 L221 L12 L213 L214 | L12 L214 L215 L216 | L114 S41 S42 S39 S40 L110 L111 L112 L4 | L4 L112 L113 L114 | L36 L37 L38 L7 | L7 L38 L1 L36 | L1 L38 L39 L32 S0 S1 S2 L33 L34 S3 S4 S5 L35 L36 | L86 L8 L15 L90 L91 L2 | L2 L91 S29 L7 S28 L86 | L39 L40 L43 L32 L7 | L7 L32 L1 L39 | L86 L16 L13 L8 | L7 S29 L1 S28 | L13 L16 L9 L8 | L86 L87 L13 L16 | L171 L172 L173 L5 L167 L168 L169 | L5 L169 L170 L171 | L41 L42 L43 L32 L44 L45 L46 L47 L7 | L7 L47 L1 L41 | L43 L40 L32 | L15 L9 L87 L88 L89 L79 L80 L81 L6 L92 L90 | S23 L1 S24 L7 | L7 S24 S25 L76 L77 L74 L75 S22 S23 | L1 S29 L92 L6 L81 L82 L83 L84 L85 S28 | L13 L87 L9 L16 | L109 L9 L104 L13 | L13 L104 L105 S30 S38 L108 L109 | L1 L47 L48 L41 | S23 S20 S21 L71 L72 L73 L74 L1 L77 L78 S26 S27 S24 | L109 L103 L104 L9 | L5 L173 L166 L167 | L50 L51 S8 S9 L7 S16 S17 L56 L57 | L7 L57 L1 L50 | L77 L1 L74 L7 | L97 L98 L99 L13 | L13 L99 L9 L97 | S30 L9 S38 L13 | L1 L57 L58 S18 S19 S16 S9 S10 L52 S11 S6 S7 L49 L50 | S121 S118 S119 L6 | L6 S119 L204 L205 L5 L207 L208 S120 S121 | L9 L99 L100 L102 L93 L94 L95 L96 L97 | S30 S31 S32 S33 S34 L106 L107 S35 S36 S37 S38 L9 | L177 L178 S84 S85 S82 S83 L174 L175 L5 | L5 L175 L176 L177 | L7 S9 L1 S16 | L63 L1 L59 L7 | L7 L59 L60 L61 L62 L63 | L100 L101 L102 L13 | L13 L102 L9 L100 | L63 L64 L65 L66 L67 L68 L69 L70 L59 L1 | S94 S95 S96 S97 S90 S91 L5 S103 S98 S99 S100 S101 S102 | L5 S102 S103 S91 S92 S93 S94 | L205 L206 L207 L5 | L200 L201 L202 L203 L192 L5 | L5 L192 L193 L194 L195 L196 L197 L198 L199 L200 | L12 L221 L212 L213 | L183 L184 S106 S107 S108 L185 S109 S104 L5 S112 S113 S110 S111 L186 L187 | L5 L187 L188 S112 S104 S105 L182 L183 | L12 L228 L222 L223 | L118 L119 L120 L121 L122 L123 L124 L125 | S47 S48 S49 S50 L129 L130 S51 S52 S53 S54 S55 L131 L132 L133 S56 S57 S58 S59 S60 L134 L135 S61 S62 S63 S64 L136 S65 | S66 S67 L137 L138 L139 L140 L141 S68 S69 | L145 L146 L147 L148 L149 L150 L151 L152 | S74 S75 L156 L157 L158 L159 L160 L161 L162 S76 S77
